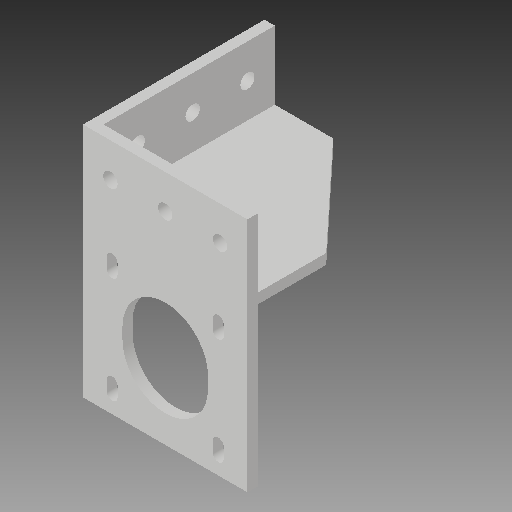
# Autodesk Inventor part: MotorMount1
Saved by Autodesk Inventor 2018 (Build 220112000, 112)
## iProperties
Created: 2017-10-01
Part Number: MotorMount1
Material: Generic
Document SubType Name: Modeling
Designer: Jurjen
Density: 1 g/cm^3
Appearance: Default
Author: Jurjen
Autodesk Inventor part; units mm, degrees
ref_plane "YZ Plane" through (0, 0, 0) normal (1, 0, 0) x (0, 1, 0)
ref_plane "XZ Plane" through (0, 0, 0) normal (0, 1, 0) x (-1, 0, 0)
ref_plane "XY Plane" through (0, 0, 0) normal (0, 0, 1) x (1, 0, 0)
sketch "Sketch1" plane through (0, 0, 0) normal (0, 0, 1) x (1, 0, 0)
  line L0 (-24, 11.5) -> (-24, -11.5)
  line L1 (-24, -11.5) -> (24, -11.5) construction
  line L2 (24, -11.5) -> (24, 11.5)
  line L3 (24, 11.5) -> (-1, 11.5)
  line L4 (-1, 11.5) -> (-24, 11.5)
  line L5 (-24, -11.5) -> (-24, -57.5)
  line L6 (-24, -57.5) -> (24, -57.5)
  line L7 (24, -57.5) -> (24, -11.5)
  point P0 (0, 0)
  point P1 (0, -11.5)
  point P2 (-24, 0)
  point P3 (11.5, 11.5)
  dimension "d0" = 23
  dimension "d1" = 23
  dimension "d2" = 48
  dimension "d6" = 48
  dimension "d7" = 46
  constraints: 16 end point, 3 midpoint, 2 horizontal alignment, 2 perpendicular, 1 horizontal, 1 parallel, 1 point on line, 1 vertical, 1 vertical alignment
  measures "d0" distance of L3.end L0.start
  measures "d1" distance of L1.end L2.end
  measures "d2" distance of L0.end L1.end
  measures "d6" distance of L5.end L6.end
  measures "d7" distance of L0.end L5.end
extrude "Extrusion1" add sketch "Sketch1" along normal mid plane 3
sketch "Sketch2" plane through (0, 0, 1.5) normal (0, 0, 1) x (1, 0, 0)
  arc A0 (-17.1, -52.5) -> (-13.9, -52.5) centre (-15.5, -52.5) ccw
  arc A1 (-13.9, -18.5) -> (-17.1, -18.5) centre (-15.5, -18.5) ccw
  arc A2 (17.1, -18.5) -> (13.9, -18.5) centre (15.5, -18.5) ccw
  arc A3 (13.9, -52.5) -> (17.1, -52.5) centre (15.5, -52.5) ccw
  arc A4 (-17.1, -21.5) -> (-13.9, -21.5) centre (-15.5, -21.5) ccw
  arc A5 (-13.9, -49.5) -> (-17.1, -49.5) centre (-15.5, -49.5) ccw
  arc A6 (13.9, -21.5) -> (17.1, -21.5) centre (15.5, -21.5) ccw
  arc A7 (17.1, -49.5) -> (13.9, -49.5) centre (15.5, -49.5) ccw
  line L0 (-17.1, -52.5) -> (-17.1, -49.5)
  line L1 (-13.9, -52.5) -> (-13.9, -49.5)
  line L2 (-17.1, -21.5) -> (-17.1, -18.5)
  line L3 (-13.9, -18.5) -> (-13.9, -21.5)
  line L4 (13.9, -18.5) -> (13.9, -21.5)
  line L5 (17.1, -21.5) -> (17.1, -18.5)
  line L6 (13.9, -49.5) -> (13.9, -52.5)
  line L7 (17.1, -52.5) -> (17.1, -49.5)
  line L8 (-24, 11.5) -> (-24, -57.5) projected
  line L9 (-24, -57.5) -> (24, -57.5) projected
  line L10 (-17.1, -51) -> (-13.9, -51) construction
  line L11 (-17.1, -20) -> (-13.9, -20) construction
  point P0 (0, 0)
  dimension "d8" = 3.2
  dimension "d9" = 3
  dimension "d10" = 8.5
  dimension "d11" = 5
  dimension "d12" = 31
  dimension "d13" = 31
  dimension "d14" = 3
  constraints: 20 end point, 16 point on circle, 8 centre point, 8 point on line, 7 equal radius, 6 tangent, 4 horizontal alignment, 4 midpoint, 3 parallel, 2 vertical alignment, 1 vertical
  measures "d8" diameter of A0
  measures "d9" distance of L0.start L0.end
  measures "d10" distance from line of L8 A0.centre
  measures "d11" distance from line of L9 A0.centre
  measures "d12" distance of A3.centre A0.centre
  measures "d13" distance between parallel lines of L11 L10
  measures "d14" distance of L2.start L2.end
extrude "Extrusion2" cut sketch "Sketch2" against normal up to next
sketch "Sketch3" plane through (0, 0, 1.5) normal (0, 0, 1) x (1, 0, 0)
  line L0 (24, 11.5) -> (24, -57.5) projected
  line L1 (24, 11.5) -> (-24, 11.5) construction
  line L2 (-24, -57.5) -> (-24, 11.5) projected
  line L3 (24, 11.5) -> (24, -57.5) projected
  line L4 (24, -57.5) -> (24, 11.5) projected
  line L5 (-24, 11.5) -> (24, 11.5) projected
  circle A0 centre (16, 1.5) radius 2.1
  circle A1 centre (0, 1.5) radius 2.1
  circle A2 centre (-16, 1.5) radius 2.1
  point P0 (0, 0)
  point P1 (35, -11.5)
  point P2 (16.6018, 1.5)
  dimension "d19" = 4.2
  dimension "d20" = 16
  dimension "d21" = 8
  dimension "d23" = 16
  dimension "d52" = 10
  constraints: 3 centre point, 3 horizontal alignment, 2 end point, 2 equal radius, 1 horizontal, 1 point on line, 3 other
  measures "d19" diameter of A0
  measures "d20" distance of A1.centre A0.centre
  measures "d23" distance of A1.centre A2.centre
  measures "d52" distance from line of L1 A0.centre
sketch "Sketch4" plane through (0, 0, -1.5) normal (0, 0, -1) x (-1, 0, 0)
  line L0 (13.9, -21.5) -> (13.9, -18.5) projected
  arc A0 (17.1, -18.5) -> (13.9, -18.5) centre (15.5, -18.5) ccw projected
  line L1 (17.1, -18.5) -> (17.1, -21.5) projected
  arc A1 (13.9, -21.5) -> (17.1, -21.5) centre (15.5, -21.5) ccw projected
  arc A2 (13.9, -52.5) -> (17.1, -52.5) centre (15.5, -52.5) ccw projected
  line L2 (13.9, -52.5) -> (13.9, -49.5) projected
  arc A3 (17.1, -49.5) -> (13.9, -49.5) centre (15.5, -49.5) ccw projected
  line L3 (17.1, -49.5) -> (17.1, -52.5) projected
  line L4 (-17.1, -52.5) -> (-17.1, -49.5) projected
  arc A4 (-13.9, -49.5) -> (-17.1, -49.5) centre (-15.5, -49.5) ccw projected
  line L5 (-13.9, -49.5) -> (-13.9, -52.5) projected
  arc A5 (-17.1, -52.5) -> (-13.9, -52.5) centre (-15.5, -52.5) ccw projected
  line L6 (-17.1, -21.5) -> (-17.1, -18.5) projected
  arc A6 (-13.9, -18.5) -> (-17.1, -18.5) centre (-15.5, -18.5) ccw projected
  line L7 (-13.9, -18.5) -> (-13.9, -21.5) projected
  arc A7 (-17.1, -21.5) -> (-13.9, -21.5) centre (-15.5, -21.5) ccw projected
  line L8 (24, -57.5) -> (24, 11.5) projected
  line L9 (24, 11.5) -> (-24, 11.5) projected
  line L10 (-24, 11.5) -> (-24, -57.5) projected
  line L11 (-24, -57.5) -> (24, -57.5) projected
  line L12 (-24, 11.5) -> (-24, -11.5) projected
  line L13 (-24, -11.5) -> (24, -11.5)
  line L14 (24, -57.5) -> (24, 11.5) projected
  line L15 (24, -8.5) -> (-24, -8.5)
  point P0 (0, 0)
  point P1 (-35, -11.5)
  dimension "d30" = 3
  constraints: 4 end point, 4 point on line, 2 perpendicular
  measures "d30" distance between parallel lines of L13 L15
extrude "Extrusion4" add sketch "Sketch4" along normal blind 50 contours L13 L10 L15 L8
sketch "Sketch8" plane through (0, 0, 1.5) normal (0, 0, 1) x (1, 0, 0)
  arc A0 (12.5, -34) -> (-12.5, -34) centre (0, -34) ccw
  arc A1 (-12.5, -37) -> (12.5, -37) centre (0, -37) ccw
  line L0 (13.9, -21.5) -> (13.9, -18.5) projected
  line L1 (13.9, -20) -> (-13.9, -20) construction
  line L2 (-13.9, -18.5) -> (-13.9, -21.5) projected
  line L3 (-13.9, -20) -> (-13.9, -51) construction
  line L4 (-13.9, -49.5) -> (-13.9, -52.5) projected
  line L5 (12.5, -34) -> (12.5, -37)
  line L6 (-12.5, -34) -> (-12.5, -37)
  point P0 (0, 0)
  point P1 (-12.5, -35.5)
  point P2 (-13.9, -35.5)
  point P3 (0, -21.5)
  point P4 (0, -20)
  dimension "d46" = 25
  dimension "d47" = 3
  constraints: 8 end point, 6 midpoint, 5 point on circle, 2 centre point, 2 tangent, 1 equal radius, 1 horizontal alignment, 1 parallel, 1 vertical, 1 vertical alignment
  measures "d46" diameter of A0
  measures "d47" distance of L5.end L5.start
extrude "Extrusion8" cut sketch "Sketch8" against normal up to next
sketch "Sketch9" plane through (-24, -57.5, 1.5) normal (-1, 0, 0) x (0, 0, 1)
  line L0 (-3, 69) -> (-3, 49) projected
  line L1 (-3, 69) -> (-53, 69)
  line L2 (-3, 49) -> (-53, 49) projected
  line L3 (-53, 46) -> (-53, 49) projected
  line L4 (-53, 69) -> (-53, 49)
  point P0 (-1.5, 57.5)
  point P1 (-53, 0)
  constraints: 4 end point, 1 horizontal, 1 vertical
extrude "Extrusion9" add sketch "Sketch9" against normal blind 3
extrude "Extrusion10" cut sketch "Sketch3" against normal up to next
sketch "Sketch10" plane through (-24, -11.5, -1.5) normal (0, -1, 0) x (1, 0, 0)
  line L0 (48, 0) -> (48, -50) projected
  line L1 (48, -20) -> (20, -50)
  line L2 (48, 0) -> (0, 0) projected
  line L3 (0, 0) -> (0, -50) projected
  line L4 (48, -50) -> (0, -50) projected
  point P0 (24, 1.5)
  dimension "d55" = 20
  dimension "d56" = 20
  constraints: 2 end point, 1 horizontal alignment, 1 point on line
  measures "d55" distance from line of L2 L1.start
  measures "d56" distance from line of L3 L1.end
extrude "Extrusion11" cut sketch "Sketch10" against normal up to next contours L0 L4 L1
sketch "Sketch11" plane through (-24, -57.5, 1.5) normal (-1, 0, 0) x (0, 0, 1)
  circle A0 centre (-13, 59) radius 2.1
  circle A1 centre (-45, 59) radius 2.1
  circle A2 centre (-29, 59) radius 2.1
  line L0 (0, 69) -> (0, 0) projected
  line L1 (0, 69) -> (-53, 69) projected
  point P0 (-1.5, 57.5)
  dimension "d59" = 4.2
  dimension "d60" = 16
  dimension "d61" = 13
  dimension "d62" = 16
  dimension "d65" = 10
  constraints: 3 centre point, 2 equal radius, 2 horizontal alignment
  measures "d59" diameter of A0
  measures "d60" distance of A0.centre A2.centre
  measures "d61" distance from line of A0.centre L0
  measures "d62" distance of A2.centre A1.centre
  measures "d65" distance from line of A0.centre L1
extrude "Extrusion12" cut sketch "Sketch11" against normal up to next
body "Solid1"
